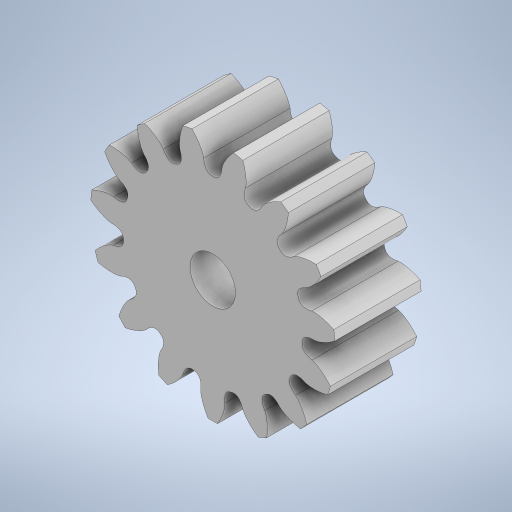
# Autodesk Inventor part: pinion_gear_mid
Saved by Autodesk Inventor 2023 (Build 270158000, 158)
## iProperties
Created: 2022-11-17
Part Number: pinion_gear_mid
Material: Generic
Document SubType Name: Modeling
Designer: eahil
Density: 1 g/cm^3
Appearance: Default
Author: eahil
Autodesk Inventor part; units mm, degrees
ref_plane "YZ Plane" through (0, 0, 0) normal (1, 0, 0) x (0, 1, 0)
ref_plane "XZ Plane" through (0, 0, 0) normal (0, 1, 0) x (-1, 0, 0)
ref_plane "XY Plane" through (0, 0, 0) normal (0, 0, 1) x (1, 0, 0)
sketch "Sketch1" plane through (0, 0, 0) normal (0, 0, 1) x (1, 0, 0)
  spline S0 degree 3 poles (-2.89, 16.7526) (-2.7988, 16.6553) (-2.6164, 16.4608) (-2.36, 16.1536) (-2.1179, 15.8352) (-1.8932, 15.5042) (-1.6884, 15.1604) (-1.5377, 14.8629) (-1.4321, 14.618) (-1.3624, 14.4306) (-1.3014, 14.2398) (-1.277, 14.1087) (-1.2648, 14.0432) knots 0 0 0 0 0.039989 0.079978 0.119966 0.159954 0.19994 0.239923 0.259918 0.279912 0.299904 0.319886 0.319886 0.319886 0.319886
  spline S1 degree 3 poles (-1.2648, 14.0432) (-1.2587, 13.9491) (-1.2495, 13.8079) (-1.2211, 13.6214) (-1.1899, 13.4834) (-1.1519, 13.3471) (-1.1014, 13.2149) (-1.0426, 13.0861) (-0.9699, 12.9645) (-0.8849, 12.8512) (-0.7866, 12.749) (-0.6756, 12.6608) (-0.5532, 12.589) (-0.4213, 12.5367) (-0.2829, 12.505) (-0.1413, 12.498) (0, 12.501) (0.1413, 12.498) (0.2829, 12.505) (0.4213, 12.5367) (0.5532, 12.589) (0.6756, 12.6608) (0.7866, 12.749) (0.8849, 12.8512) (0.9699, 12.9645) (1.0426, 13.0861) (1.1014, 13.2149) (1.1519, 13.3471) (1.1899, 13.4834) (1.2211, 13.6214) (1.2495, 13.8079) (1.2587, 13.9491) (1.2648, 14.0432) knots 0 0 0 0 0.028272 0.042412 0.05655 0.070691 0.084827 0.098966 0.113106 0.127244 0.141379 0.155515 0.169653 0.183788 0.197919 0.212046 0.226186 0.240326 0.254453 0.268584 0.282719 0.296857 0.310993 0.325128 0.339266 0.353406 0.367545 0.381681 0.395822 0.40996 0.4241 0.452372 0.452372 0.452372 0.452372
  spline S2 degree 3 poles (1.2648, 14.0432) (1.277, 14.1087) (1.3014, 14.2398) (1.3624, 14.4306) (1.4321, 14.618) (1.5377, 14.8629) (1.6884, 15.1604) (1.8932, 15.5042) (2.1179, 15.8352) (2.36, 16.1536) (2.6164, 16.4608) (2.7988, 16.6553) (2.89, 16.7526) knots 0 0 0 0 0.019982 0.039974 0.059968 0.079963 0.119946 0.159932 0.19992 0.239909 0.279898 0.319886 0.319886 0.319886 0.319886
  circle A0 centre (0, 0) radius 12.5 construction
  circle A1 centre (0, 0) radius 14.0954 construction
  circle A2 centre (0, 0) radius 15 construction
  circle A3 centre (0, 0) radius 17
  point P0 (-2.6192, 16.4582)
  point P1 (-2.3624, 16.1517)
  point P2 (-2.1208, 15.8331)
  point P3 (-1.8965, 15.502)
  point P4 (-1.6924, 15.1582)
  point P5 (-1.5126, 14.8011)
  point P6 (-1.4337, 14.6174)
  point P7 (-1.3639, 14.43)
  point P8 (-1.3054, 14.2388)
  point P9 (-1.241, 13.7614)
  point P10 (-1.2194, 13.6217)
  point P11 (-1.1888, 13.4837)
  point P12 (-1.1498, 13.3478)
  point P13 (-1.1, 13.2154)
  point P14 (-1.0403, 13.0873)
  point P15 (-0.9679, 12.9659)
  point P16 (-0.8827, 12.853)
  point P17 (-0.7845, 12.7513)
  point P18 (-0.6737, 12.6636)
  point P19 (-0.5516, 12.5923)
  point P20 (-0.4202, 12.5401)
  point P21 (-0.2823, 12.5091)
  point P22 (-0.1414, 12.4997)
  point P23 (0, 12.5)
  point P24 (0.1414, 12.4997)
  point P25 (0.2823, 12.5091)
  point P26 (0.4202, 12.5401)
  point P27 (0.5516, 12.5923)
  point P28 (0.6737, 12.6636)
  point P29 (0.7845, 12.7513)
  point P30 (0.8827, 12.853)
  point P31 (0.9679, 12.9659)
  point P32 (1.0403, 13.0873)
  point P33 (1.1, 13.2154)
  point P34 (1.1498, 13.3478)
  point P35 (1.1888, 13.4837)
  point P36 (1.2194, 13.6217)
  point P37 (1.241, 13.7614)
  point P38 (1.3054, 14.2388)
  point P39 (1.3639, 14.43)
  point P40 (1.4337, 14.6174)
  point P41 (1.5126, 14.8011)
  point P42 (1.6924, 15.1582)
  point P43 (1.8965, 15.502)
  point P44 (2.1208, 15.8331)
  point P45 (2.3624, 16.1517)
  point P46 (2.6192, 16.4582)
  constraints: 4 centre point, 2 point on circle, 109 other
extrude "Extrusion1" add sketch "Sketch1" against normal blind 12
extrude "Extrusion2" cut sketch "Sketch1" against normal through all contours A3 S2 S1 S0 picked at (0.2965, 15.5213)
pattern_circular "Circular Pattern2" count 15 over 360 about axis through (0, 0, -10) along (0, 0, 1) of "Extrusion2"
sketch "Sketch2" plane through (0, 0, 0) normal (0, 0, 1) x (1, 0, 0)
  point P0 (0, 0)
  point P1 (0, 0)
  constraints: 1 coincident
hole "Hole1" at (0, 0, 0) direction (0, 0, -1) diameter 6.32 end through all
equation "\"d0\" = FaceWidth"
equation "\"Module\" = 2"
equation "\"PressureAngle\" = 20deg"
equation "\"UnitProfileClearance\" = 0.25"
equation "\"UnitRoundRadius\" = 0.35"
equation "\"HeadDiameter\" = 34"
equation "\"RootDiameter\" = 25"
equation "\"BaseDiameter\" = 28.19078"
equation "\"FaceWidth\" = 12"
equation "\"HelixAngle\" = 0"
equation "\"UnitCorrection\" = 0"
equation "\"UnitAddendumModification\" = 0"
equation "\"CircularPitch\" = 6.283185"
equation "\"UnitBacklashShift\" = 0"
equation "\"TotalToolShift\" = 0"
equation "\"IsInternal\" = 0"
body "Solid1"
